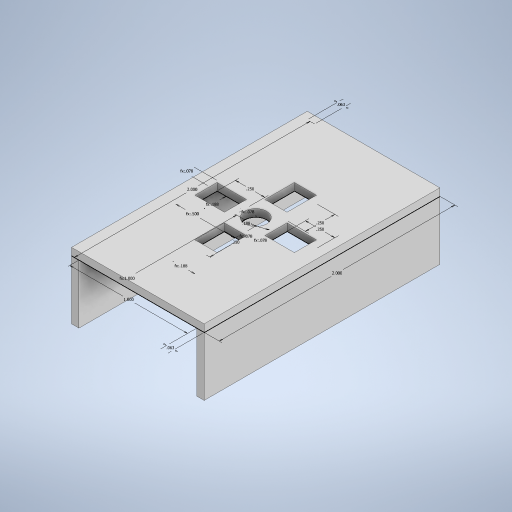
# Autodesk Inventor part: Guide for 2in box tube 1side
Saved by Autodesk Inventor 2023 (Build 270158000, 158)
## iProperties
Created: 2023-01-21
Part Number: Guide for 2in box tube 1side
Material: Generic
Document SubType Name: Modeling
Designer: Gabriel - T3 CAD
Density: 1 g/cm^3
Appearance: Default
Author: Gabriel - T3 CAD
Autodesk Inventor part; units mm, degrees
ref_plane "YZ Plane" through (0, 0, 0) normal (1, 0, 0) x (0, 1, 0)
ref_plane "XZ Plane" through (0, 0, 0) normal (0, 1, 0) x (-1, 0, 0)
ref_plane "XY Plane" through (0, 0, 0) normal (0, 0, 1) x (1, 0, 0)
sketch "Sketch1" plane through (0, 0, 0) normal (0, 1, 0) x (-1, 0, 0)
  line L0 (0, 0) -> (25.4, 0)
  line L1 (25.4, 0) -> (25.4, 50.8)
  line L2 (25.4, 50.8) -> (0, 50.8)
  line L3 (0, 50.8) -> (0, 0)
  line L4 (0, 0) -> (-1.5875, 0)
  line L5 (-1.5875, 0) -> (-1.5875, 50.8)
  line L6 (-1.5875, 50.8) -> (0, 50.8)
  line L7 (0, 50.8) -> (0, 0)
  line L8 (25.4, 50.8) -> (26.9875, 50.8)
  line L9 (26.9875, 50.8) -> (26.9875, 0)
  line L10 (26.9875, 0) -> (25.4, 0)
  line L11 (25.4, 0) -> (25.4, 50.8)
  line L12 (25.4, 27.7812) -> (0, 27.7812)
  line L13 (0, 27.7812) -> (0, 23.0187)
  line L14 (0, 23.0187) -> (25.4, 23.0188)
  line L15 (25.4, 23.0188) -> (25.4, 27.7812)
  line L16 (15.0812, 50.8) -> (10.3187, 50.8)
  line L17 (10.3187, 50.8) -> (10.3187, 0)
  line L18 (10.3187, 0) -> (15.0812, 0)
  line L19 (15.0812, 0) -> (15.0812, 50.8)
  circle A0 centre (12.7, 25.4) radius 2.3813
  line L20 (8.3344, 27.7812) -> (1.9844, 27.7812)
  line L21 (1.9844, 27.7812) -> (1.9844, 23.0187)
  line L22 (1.9844, 23.0187) -> (8.3344, 23.0187)
  line L23 (8.3344, 23.0187) -> (8.3344, 27.7812)
  line L24 (23.4156, 27.7812) -> (17.0656, 27.7812)
  line L25 (17.0656, 27.7812) -> (17.0656, 23.0187)
  line L26 (17.0656, 23.0187) -> (23.4156, 23.0188)
  line L27 (23.4156, 23.0188) -> (23.4156, 27.7812)
  line L28 (15.0812, 36.1156) -> (10.3187, 36.1156)
  line L29 (10.3187, 36.1156) -> (10.3187, 29.7656)
  line L30 (10.3187, 29.7656) -> (15.0812, 29.7656)
  line L31 (15.0812, 29.7656) -> (15.0812, 36.1156)
  line L32 (15.0812, 21.0344) -> (10.3187, 21.0344)
  line L33 (10.3187, 21.0344) -> (10.3187, 14.6844)
  line L34 (10.3187, 14.6844) -> (15.0812, 14.6844)
  line L35 (15.0812, 14.6844) -> (15.0812, 21.0344)
  point P0 (12.7, 36.1156)
  point P1 (0, 50.8)
  point P2 (1.9844, 27.7812)
  point P3 (0, 50.8)
  dimension "d0" = 25.4
  dimension "d1" = 50.8
  dimension "d2" = 1.5875
  dimension "d3" = 50.8
  dimension "d4" = 1.5875
  dimension "d5" = 4.7625
  dimension "d6" = 4.7625
  dimension "d7" = 4.7625
  dimension "d8" = 25.4
  dimension "d9" = 12.7
  dimension "d10" = 6.35
  dimension "d11" = 6.35
  dimension "d12" = 6.35
  dimension "d13" = 1.9844
  dimension "d14" = 1.9844
  dimension "d15" = 1.9844
  dimension "d16" = 1.9844
  dimension "d17" = 6.35
  constraints: 72 end point, 18 parallel, 13 point on line, 9 horizontal, 9 perpendicular, 2 tangent, 1 centre point, 1 midpoint
  measures "d0" distance of L2.end L1.end
  measures "d1" distance of L1.end L0.end
  measures "d2" distance of L5.end L6.end
  measures "d3" distance of L4.end L5.end
  measures "d4" distance of L9.end L10.end
  measures "d5" distance between parallel lines of L19 L17
  measures "d6" distance between parallel lines of L14 L12
  measures "d7" diameter of A0
  measures "d8" distance from line of L2 A0.centre
  measures "d9" distance from line of L1 A0.centre
  measures "d10" distance of L22.end L21.end
  measures "d11" distance of L26.end L25.end
  measures "d12" distance of L33.end L32.end
  measures "d13" distance between parallel lines of L17 L23
  measures "d14" distance between parallel lines of L19 L25
  measures "d15" distance between parallel lines of L12 L30
  measures "d16" distance between parallel lines of L14 L32
  measures "d17" distance from line of L30 point (12.7, 36.116)
extrude "Extrusion1" add sketch "Sketch1" along normal blind 1.5875 contours L3 L14 L17 L0 | L4 L5 L6 L3 | L17 L34 L19 L0 | L3 L12 L21 L14 | L19 L14 L1 L0 | L3 L2 L17 L12 | L1 L8 L9 L10 | L17 L14 L19 L32 | L23 L12 L17 L14 | L14 L27 L12 L1 | L17 A0 L14 | L2 L19 L28 L17 | L12 L19 L2 L1 | L19 L12 L25 L14 | L14 A0 L19 | L17 L12 A0 | L17 L30 L19 L12 | A0 L12 L19
extrude "Extrusion2" add sketch "Sketch1" against normal blind 12.7 contours L4 L5 L6 L3 | L1 L8 L9 L10
equation "\"d5\" = d7"
equation "\"d6\" = d7"
equation "\"d8\" = 0.5 * d3"
equation "\"d9\" = 0.5 * d0"
equation "\"d13\" = -0.25 * d7 + 0.25 * d0 - 0.5 * d11"
equation "\"d14\" = d13"
equation "\"d15\" = d14"
equation "\"d16\" = d14"
body "Solid1"
